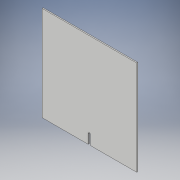
# Autodesk Inventor part: mask template
Saved by Autodesk Inventor 2017 (Build 210142000, 142)
## iProperties
Created: 2016-12-03
Part Number: mask template
Material: Generic
Document SubType Name: Modeling
Designer: Darien Morrow
Density: 1 g/cm^3
Appearance: Default
Author: Darien Morrow
Autodesk Inventor part; units mm, degrees
ref_plane "YZ Plane" through (0, 0, 0) normal (1, 0, 0) x (0, 1, 0)
ref_plane "XZ Plane" through (0, 0, 0) normal (0, 1, 0) x (-1, 0, 0)
ref_plane "XY Plane" through (0, 0, 0) normal (0, 0, 1) x (1, 0, 0)
sketch "Sketch1" plane through (0, 0, 0) normal (0, 0, 1) x (1, 0, 0)
  line L0 (-63.5, -63.5) -> (63.5, -63.5)
  line L1 (63.5, -63.5) -> (63.5, 63.5)
  line L2 (63.5, 63.5) -> (-63.5, 63.5)
  line L3 (-63.5, 63.5) -> (-63.5, -63.5)
  line L4 (-63.5, -63.5) -> (63.5, 63.5) construction
  line L5 (63.5, -63.5) -> (-63.5, 63.5) construction
  point P0 (0, 0)
  dimension "d0" = 127
  dimension "d1" = 127
  constraints: 12 end point, 2 midpoint, 2 parallel, 1 horizontal, 1 perpendicular
  measures "d0" distance between parallel lines of L1 L3
  measures "d1" distance between parallel lines of L0 L2
extrude "Extrusion1" add sketch "Sketch1" along normal blind 1.5875
sketch "Sketch2" plane through (0, 0, 0) normal (0, 0, -1) x (-1, 0, 0)
  line L0 (0, -76.2) -> (0, -50.8) construction
  line L1 (63.5, -63.5) -> (-63.5, -63.5) projected
  line L2 (1.5875, -76.2) -> (1.5875, -50.8)
  line L3 (-1.5875, -50.8) -> (-1.5875, -76.2)
  arc A0 (-1.5875, -76.2) -> (1.5875, -76.2) centre (0, -76.2) ccw
  arc A1 (1.5875, -50.8) -> (-1.5875, -50.8) centre (0, -50.8) ccw
  point P0 (0, 0)
  point P1 (0, -63.5)
  dimension "d4" = 12.7
  dimension "d5" = 3.175
  constraints: 8 end point, 4 point on circle, 4 tangent, 2 centre point, 2 midpoint, 1 parallel, 1 vertical
  measures "d4" distance of point (0, -63.5) L0.end
  measures "d5" diameter of A1
extrude "Extrusion2" cut sketch "Sketch2" against normal blind 1.5875
body "Solid1"
